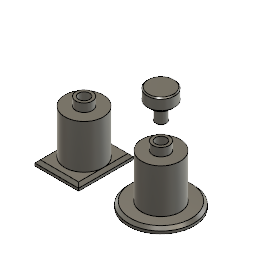
YIS805 Z80 Board Holder (Autodesk Fusion 360 design; units mm, degrees)
Autodesk Fusion 360 part; units mm, degrees
cylinder "CylinderPrimitive1" add diameter 12 height 1 placed x (1, 0, 0) y (0, 0, -1) z (0, 1, 0) at (0, 0, 0) makes body 1
cylinder "CylinderPrimitive2" add diameter 7 height 10 placed x (1, 0, 0) y (0, 0, -1) z (0, 1, 0) at (0, 1, 0) bodies 1
cylinder "CylinderPrimitive3" add diameter 3 height 1.5 placed x (1, 0, 0) y (0, 0, -1) z (0, 1, 0) at (0, 11, 0) bodies 1
cylinder "CylinderPrimitive4" cut diameter 2 height -11 placed x (1, 0, 0) y (0, 0, -1) z (0, 1, 0) at (0, 12.5, 0) bodies 1
chamfer "Chamfer1" distance 0.5 angle 45 1 edges at (-5.594, 1, 2.1697) on bodies 1
cylinder "CylinderPrimitive5" add diameter 2 height 3 placed x (1, 0, 0) y (0, 0, -1) z (0, 1, 0) at (0, 12.5, 0) separate body makes body 2
chamfer "Chamfer2" distance 0.25 angle 45 1 edges at (-0.9323, 12.5, -0.3616) on bodies 2
move_body "Move1" bodies 2 to x (1, 0, 0) y (0, 1, 0) z (0, 0, 1) at (0, 1, 0)
cylinder "CylinderPrimitive6" add diameter 5 height 2.5 placed x (1, 0, 0) y (0, 0, -1) z (0, 1, 0) at (0, 16.5, 0) separate body makes body 3
chamfer "Chamfer3" distance 0.5 angle 45 1 edges at (-2.3308, 16.5, -0.904) on bodies 3
chamfer "Chamfer4" distance 0.2 angle 45 1 edges at (-2.3308, 19, 0.904) on bodies 3
combine "Combine1" operation add target body 3 tool bodies 2
copy_body "CopyPasteBodies1" bodies 1 makes body 4
move_body "Move2" bodies 4 to x (1, 0, 0) y (0, 1, 0) z (0, 0, 1) at (-14, 0, 0)
extrude "Extrude1" cut 1 faces at (-14.6642, 0, -0.4961) along direction (0, 1, 0) blind 1 on bodies 4 bodies 4
box "BoxPrimitive1" add length 10 width 8 height 1 placed x (0, 0, -1) y (1, 0, 0) z (0, -1, 0) at (-18, 1, 4) separate body makes body 5
move_body "Move3" bodies 5 to x (1, 0, 0) y (0, 1, 0) z (0, 0, 1) at (0, 0, 1)
chamfer "Chamfer5" distance 0.5 angle 45 4 edges at (-10, 1, 0) (-14, 1, 5) (-18, 1, 0) (-14, 1, -5) on bodies 5
combine "Combine2" operation add target body 4 tool bodies 5
extrude "Extrude2" cut 2 faces at (-11.1853, 11, 0.2484) (2.8147, 11, 0.2484) along direction (0, -1, 0) blind 2 on bodies 1 4 bodies 1 4
extrude "Extrude3" cut 2 faces at (-12.676, 12.5, 0.1242) (1.324, 12.5, 0.1242) along direction (0, -1, 0) blind 2 on bodies 1 4 bodies 1 4
named bodies: "BoardHolder1", "Pin", "BoardHolder", "BoardHolder2"
